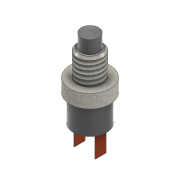
# Autodesk Inventor part: Interruptor_BlueRobotics
Saved by Autodesk Inventor 2022.3 (Build 263350000, 350)
## iProperties
Created: 2023-07-17
Part Number: Interruptor_BlueRobotics
Material: Genérico
Document SubType Name: Modeling
Designer: Usuario
Density: 1 g/cm^3
Appearance: Valor por defecto
Author: Usuario
Autodesk Inventor part; units mm, degrees
ref_plane "YZ Plane" through (0, 0, 0) normal (1, 0, 0) x (0, 1, 0)
ref_plane "XZ Plane" through (0, 0, 0) normal (0, 1, 0) x (-1, 0, 0)
ref_plane "XY Plane" through (0, 0, 0) normal (0, 0, 1) x (1, 0, 0)
sketch "Boceto1" plane through (0, 0, 0) normal (0, 1, 0) x (-1, 0, 0)
  circle A0 centre (0, 0) radius 3
  dimension "d0" = 6
  constraints: 1 centre point, 1 coincident
  measures "d0" diameter of A0
extrude "Extrusión1" add sketch "Boceto1" along normal blind 6
sketch "Boceto2" plane through (0, 6, 0) normal (0, 1, 0) x (1, 0, 0)
  circle A0 centre (0, 0) radius 2.075
  dimension "d3" = 4.15
  constraints: 1 centre point, 1 coincident
  measures "d3" diameter of A0
extrude "Extrusión2" add sketch "Boceto2" along normal blind 3.6
chamfer "Chaflán1" distance 2 distance2 0.5 1 edges at (-2.075, 9.6, 0) measured on face at (0.6845, 9.6, -0.4587)
sketch "Boceto3" plane through (0, 0, 0) normal (0, -1, 0) x (1, 0, 0)
  circle A0 centre (0, 0) radius 0.075 projected
  circle A1 centre (0, 0) radius 4.775
  dimension "d9" = 9.55
  constraints: 1 centre point, 1 coincident
  measures "d9" diameter of A1
extrude "Extrusión3" add sketch "Boceto3" along normal blind 3.2
sketch "Boceto4" plane through (0, -3.2, 0) normal (0, -1, 0) x (1, 0, 0)
  circle A0 centre (0, 0) radius 3.925
  dimension "d12" = 7.85
  constraints: 1 centre point, 1 coincident
  measures "d12" diameter of A0
extrude "Extrusión4" add sketch "Boceto4" along normal blind 6.25
thread "Rosca1" size "M6x1" class "6g" standard "ANSI Metric M Profile" length 6.2
chamfer "Chaflán2" distance 0.5 angle 45 1 edges at (3, 6, 0)
sketch "Boceto5" plane through (0, -9.45, 0) normal (0, -1, 0) x (1, 0, 0)
  circle A0 centre (0, 0) radius 0.075 projected
  line L0 (0, 0) -> (2.5, 0)
  line L1 (0, 0) -> (-2.5, 0)
  line L2 (2.45, 1.275) -> (2.55, 1.275)
  line L3 (2.55, 1.275) -> (2.55, -1.275)
  line L4 (2.55, -1.275) -> (2.45, -1.275)
  line L5 (2.45, -1.275) -> (2.45, 1.275)
  line L6 (2.45, 1.275) -> (2.55, -1.275) construction
  line L7 (2.55, 1.275) -> (2.45, -1.275) construction
  line L8 (-2.55, 1.275) -> (-2.45, 1.275)
  line L9 (-2.45, 1.275) -> (-2.45, -1.275)
  line L10 (-2.45, -1.275) -> (-2.55, -1.275)
  line L11 (-2.55, -1.275) -> (-2.55, 1.275)
  line L12 (-2.55, 1.275) -> (-2.45, -1.275) construction
  line L13 (-2.45, 1.275) -> (-2.55, -1.275) construction
  dimension "d20" = 2.5
  dimension "d21" = 2.5
  dimension "d22" = 0.1
  dimension "d23" = 2.55
  dimension "d24" = 0.1
  constraints: 28 end point, 4 horizontal, 4 midpoint, 4 parallel, 2 perpendicular, 1 point on line
  measures "d20" distance of L0.start L0.end
  measures "d21" distance of L0.start L1.end
  measures "d22" distance of L3.end L4.end
  measures "d23" distance of L2.end L3.end
  measures "d24" distance of L9.end L10.end
extrude "Extrusión5" add sketch "Boceto5" along normal blind 5.5 contours L9 L10 L11 L8 | L5 L2 L3 L4
